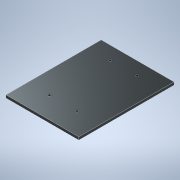
# Autodesk Inventor part: palte cylinder
Saved by Autodesk Inventor 2022.2 (Build 262287000, 287)
## iProperties
Created: 2022-02-23
Part Number: palte cylinder
Material: Iron, Gray
Document SubType Name: Modeling
Designer: ONG
Density: 7.15 g/cm^3
Appearance: Iron Gray
Author: ONG
Autodesk Inventor part; units mm, degrees
ref_plane "YZ Plane" through (0, 0, 0) normal (1, 0, 0) x (0, 1, 0)
ref_plane "XZ Plane" through (0, 0, 0) normal (0, 1, 0) x (-1, 0, 0)
ref_plane "XY Plane" through (0, 0, 0) normal (0, 0, 1) x (1, 0, 0)
sketch "Sketch1" plane through (0, 0, 0) normal (0, 1, 0) x (-1, 0, 0)
  line L0 (-130, -170) -> (130, -170)
  line L1 (130, -170) -> (130, 170)
  line L2 (130, 170) -> (-130, 170)
  line L3 (-130, 170) -> (-130, -170)
  line L4 (-130, -170) -> (130, 170) construction
  line L5 (130, -170) -> (-130, 170) construction
  point P0 (0, 0)
  dimension "d0" = 260
  dimension "d1" = 340
  constraints: 12 end point, 2 midpoint, 2 parallel, 1 horizontal, 1 perpendicular
  measures "d0" distance of L2.end L1.end
  measures "d1" distance of L1.end L0.end
extrude "Extrusion1" add sketch "Sketch1" along normal blind 10
sketch "Sketch2" plane through (0, 10, 0) normal (0, 1, 0) x (1, 0, 0)
  point P0 (-50, 122.3557)
  point P1 (44.9988, 123.5432)
  point P2 (46.7815, -93.6443)
  point P3 (-51.5466, -93.6443)
hole "Hole1" at (-50, 10, -122.3557) at (44.9988, 10, -123.5432) at (46.7815, 10, 93.6443) at (-51.5466, 10, 93.6443) direction (0, -1, 0) diameter 8.376 end through all thread size "M10x1.5" designation "M10" class "6H" standard "GB Metric profile"
body "Solid1"
